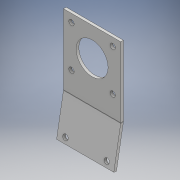
# Autodesk Inventor part: Handplatte 2
Saved by Autodesk Inventor 2017 (Build 210142000, 142)
## iProperties
Created: 2018-06-06
Part Number: Handplatte 2
Material: Generic
Document SubType Name: Sheet Metal
Designer: Zeno's Kiste
Density: 1 g/cm^3
Sheet Metal Rule: 2 mm Aluminium
Appearance: Default
Flat Pattern Width: 4.3 cm
Flat Pattern Length: 8.3 cm
Flat Pattern Area: 35.69 cm^2
Sheet Metal Width: 43,000 mm
Sheet Metal Length: 83,000 mm
Sheet Metal Area: 3569,000 mm^2
Author: Zeno's Kiste
Autodesk Inventor part; units mm, degrees
ref_plane "YZ Plane" through (0, 0, 0) normal (1, 0, 0) x (0, 1, 0)
ref_plane "XZ Plane" through (0, 0, 0) normal (0, 1, 0) x (-1, 0, 0)
ref_plane "XY Plane" through (0, 0, 0) normal (0, 0, 1) x (1, 0, 0)
sketch "Sketch1" plane through (0, 0, 0) normal (0, 1, 0) x (-1, 0, 0)
  line L0 (-21.5, 42.0075) -> (-21.5, -40.9925)
  circle A0 centre (-15.5, -36.9925) radius 2
  circle A1 centre (-15.5, 5.0075) radius 2
  circle A2 centre (-15.5, 36.0075) radius 2
  line L1 (-21.5, -40.9925) -> (0, -40.9925)
  line L2 (-21.5, 42.0075) -> (0, 42.0075)
  line L3 (0, 42.0075) -> (21.5, 42.0075)
  line L4 (21.5, 42.0075) -> (21.5, -40.9925)
  line L5 (21.5, -40.9925) -> (0, -40.9925)
  line L6 (0, -40.9925) -> (0, 42.0075) construction
  circle A3 centre (15.5, 5.0075) radius 2
  circle A4 centre (15.5, 36.0075) radius 2
  circle A5 centre (15.5, -36.9925) radius 2
  line L7 (21.5, 20.5075) -> (-21.5, 20.5075) construction
  line L8 (21.5, -10.9925) -> (-21.5, -10.9925) construction
  circle A6 centre (0, 20.5075) radius 12
  point P0 (0, 0)
  dimension "d1" = 83
  dimension "d6" = 4
  dimension "d13" = 31
  dimension "d14" = 43
  dimension "d15" = 31
  dimension "d16" = 4
  dimension "d17" = 6
  dimension "d18" = 30
  dimension "d19" = 43
  dimension "d20" = 24
  measures "d1" distance of L0.end L0.start
  measures "d6" diameter of A0
  measures "d13" distance of A1.centre A3.centre
  measures "d14" distance of L0.start L3.end
  measures "d15" distance of A2.centre A1.centre
  measures "d16" distance from line of L5 A5.centre
  measures "d17" distance from line of L4 A5.centre
  measures "d18" distance between parallel lines of L5 L8
  measures "d19" diameter of L2 L7
  measures "d20" diameter of A6
extrude "Plate1" add sketch "Sketch1" along normal blind 2
sketch "Sketch2" plane through (0, 2, 0) normal (0, 1, 0) x (1, 0, 0)
  line L0 (-21.5, -42.0075) -> (-21.5, 40.9925) projected
  line L1 (-21.5, 10.9925) -> (21.5, 10.9925)
  line L2 (21.5, 40.9925) -> (21.5, -42.0075) projected
  line L3 (-21.5, 40.9925) -> (21.5, 40.9925) projected
  point P0 (0, 0)
  dimension "d22" = 30
  constraints: 2 end point, 2 point on line, 1 horizontal
  measures "d22" distance between parallel lines of L3 L1
fold "Fold1" angle 10 bend radius 2 thickness 2 k factor 0.44 line from (-21.5, 2, -10.9925) to (21.5, 2, -10.9925) line at bend centre moving side (0, 0, -1) folds toward (0, -1, 0)
equation "\"d23\" = BendReliefWidth"
equation "\"d24\" = BendReliefDepth"
equation "\"d25\" = MinimumRemnant"
equation "\"d26\" = BendRadius"
equation "\"d28\" = BendRadius"
equation "\"BendRadius\" = Thickness"
equation "\"BendReliefWidth\" = Thickness"
equation "\"BendReliefDepth\" = 0.5 * Thickness"
equation "\"CornerReliefSize\" = 4 * Thickness"
equation "\"MinimumRemnant\" = 2 * Thickness"
equation "\"TransitionRadius\" = BendRadius"
equation "\"JacobiRadiusSize\" = BendRadius"
equation "\"GapSize\" = Thickness"
equation "\"d21\" = BendRadius"
equation "\"Thickness\" = 2"
body "Solid1"
